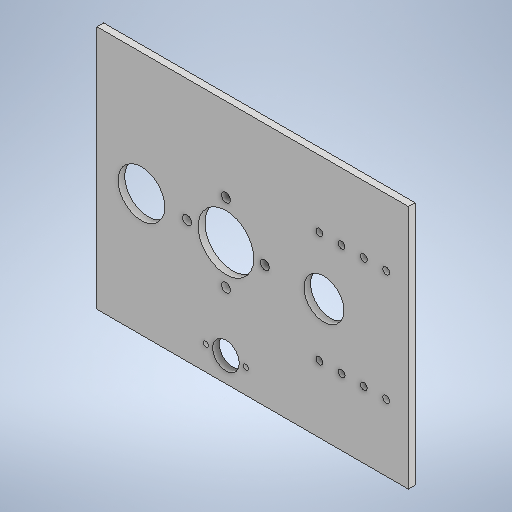
# Autodesk Inventor part: dr_plate_motor
Saved by Autodesk Inventor 2025.1 (Build 291241000, 241)
## iProperties
Created: 2025-05-01
Part Number: dr_plate_motor
Material: 一般
Document SubType Name: Modeling
Designer: yuki0520
Density: 1 g/cm^3
Appearance: 既定
Author: yuki0520
Autodesk Inventor part; units mm, degrees
ref_plane "YZ Plane" through (0, 0, 0) normal (1, 0, 0) x (0, 1, 0)
ref_plane "XZ Plane" through (0, 0, 0) normal (0, 1, 0) x (-1, 0, 0)
ref_plane "XY Plane" through (0, 0, 0) normal (0, 0, 1) x (1, 0, 0)
derived "zzz_sekkei2.ipt"
sketch "スケッチ1" plane through (0, 0, 0) normal (0, 0, 1) x (1, 0, 0)
  circle A0 centre (0, 0) radius 120
  line L0 (-120, 0) -> (120, 0)
  circle A1 centre (-158, 0) radius 38
  line L1 (-120, -55) -> (-120, 55)
  line L2 (-120, 25) -> (-165, 25)
  line L3 (-165, 25) -> (-165, -25)
  line L4 (-165, -25) -> (-120, -25)
  line L5 (-120, -25) -> (-120, 25)
  circle A2 centre (-160, 25) radius 1.55
  circle A3 centre (-150, 25) radius 1.55
  circle A4 centre (-140, 25) radius 1.55
  circle A5 centre (-160, -25) radius 1.55
  circle A6 centre (-150, -25) radius 1.55
  circle A7 centre (-140, -25) radius 1.55
  circle A8 centre (-158, 0) radius 9
  line L6 (0, -120) -> (0, 120)
  circle A9 centre (-202, 0) radius 12.5
  line L7 (-48.1437, 0) -> (-120, 0)
  circle A10 centre (-202, 0) radius 17.5
  circle A11 centre (-184.5, 0) radius 2.05
  circle A12 centre (-202, 17.5) radius 2.05
  circle A13 centre (-219.5, 0) radius 2.05
  circle A14 centre (-202, -17.5) radius 2.05
  line L8 (-260, -55) -> (-120, -55)
  line L9 (-120, -55) -> (-120, 55)
  line L10 (-120, 55) -> (-260, 55)
  line L11 (-260, 55) -> (-260, -55)
  line L12 (-260, -55) -> (-120, 55) construction
  line L13 (-120, -55) -> (-260, 55) construction
  circle A15 centre (-240, 0) radius 10.5
  circle A16 centre (-202, -44) radius 6
  circle A17 centre (-202, -44) radius 9
  circle A18 centre (-202, -53) radius 1.15
  line L14 (-202, 17.5) -> (-202, -17.5)
  circle A19 centre (-193, -44) radius 1.15
  circle A20 centre (-202, -35) radius 1.15
  circle A21 centre (-211, -44) radius 1.15
  circle A22 centre (-130, 25) radius 1.55
  circle A23 centre (-130, -25) radius 1.55
  line L15 (138.5, -104) -> (120, -104)
  line L16 (120, -104) -> (120, 104)
  line L17 (120, 104) -> (138.5, 104)
  line L18 (138.5, 104) -> (138.5, -104)
  line L19 (138.5, -104) -> (120, 104) construction
  line L20 (120, -104) -> (138.5, 104) construction
  circle A24 centre (202, -17.5) radius 2.05
  circle A25 centre (211, -44) radius 1.15
  line L21 (260, 55) -> (260, -55)
  line L22 (120, 55) -> (260, 55)
  circle A26 centre (158, 0) radius 38
  line L23 (120, -55) -> (260, 55) construction
  line L24 (260, -55) -> (120, 55) construction
  line L25 (120, -55) -> (120, 55)
  line L26 (120, -55) -> (120, 55)
  line L27 (260, -55) -> (120, -55)
  circle A27 centre (240, 0) radius 10.5
  circle A28 centre (193, -44) radius 1.15
  circle A29 centre (202, 17.5) radius 2.05
  circle A30 centre (219.5, 0) radius 2.05
  circle A31 centre (184.5, 0) radius 2.05
  circle A32 centre (160, 25) radius 1.55
  circle A33 centre (158, 0) radius 9
  circle A34 centre (160, -25) radius 1.55
  line L28 (165, 25) -> (165, -25)
  circle A35 centre (150, 25) radius 1.55
  circle A36 centre (140, 25) radius 1.55
  circle A37 centre (140, -25) radius 1.55
  line L29 (120, -25) -> (120, 25)
  line L30 (165, -25) -> (120, -25)
  circle A38 centre (150, -25) radius 1.55
  circle A39 centre (202, -53) radius 1.15
  circle A40 centre (202, 0) radius 12.5
  line L31 (202, 17.5) -> (202, -17.5)
  circle A41 centre (202, 0) radius 17.5
  circle A42 centre (202, -44) radius 6
  circle A43 centre (202, -44) radius 9
  circle A44 centre (202, -35) radius 1.15
  line L32 (120, 25) -> (165, 25)
  circle A45 centre (130, 25) radius 1.55
  circle A46 centre (130, -25) radius 1.55
  point P0 (-190, 0)
  point P1 (129.25, 0)
  point P2 (120, 0)
  point P3 (120, 0)
  point P4 (190, 0)
extrude "押し出し1" add sketch "スケッチ1" along normal blind 3 contours L1 L4 A23 A1 | A1 A23 L4 A7 A6 A5 L3 A8 L2 A2 A3 A4 A22 | A1 A22 L2 L1 | L1 L8 L11 L10 L2 A22 A1 A10 A12 A13 A14 A23 L4 | L2 A4 A3 A2 L3 A8 L4 A5 A6 A7 A23 A1 A10 A11 A22 | A10 A11 A1 A9 | A1 A9 L14 A12 A10 | A10 A14 L14 A9 A1 | A9 L14 A14 A10 A13 A12 | A19 A17 A18 A21 A20 | A20 A17 | A17 A20 | A18 A17 | A17 A18
